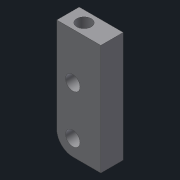
# Autodesk Inventor part: pci_slot_adapter_04
Saved by Autodesk Inventor 2022 (Build 260153000, 153)
## iProperties
Created: 2025-02-02
Part Number: pci_slot_adapter_04
Material: 一般
Document SubType Name: Modeling
Designer: nyxeon
Density: 1 g/cm^3
Appearance: 既定
Author: nyxeon
Autodesk Inventor part; units mm, degrees
ref_plane "YZ Plane" through (0, 0, 0) normal (1, 0, 0) x (0, 1, 0)
ref_plane "XZ Plane" through (0, 0, 0) normal (0, 1, 0) x (-1, 0, 0)
ref_plane "XY Plane" through (0, 0, 0) normal (0, 0, 1) x (1, 0, 0)
sketch "スケッチ1" plane through (0, 0, 0) normal (0, 0, 1) x (1, 0, 0)
  circle A0 centre (250, 70) radius 2.1 construction
  circle A1 centre (250, 85) radius 2.1 construction
  line L0 (258.724, 99.45) -> (245, 99.45) projected
  arc A2 (245, 70) -> (250, 65) centre (250, 70) ccw
  line L1 (245, 70) -> (245, 99.45)
  line L2 (258.724, 99.45) -> (258.724, 65)
  line L3 (258.724, 65) -> (250, 65)
  circle A3 centre (250, 70) radius 2.25
  circle A4 centre (250, 85) radius 2.25
  point P0 (0, 0)
  dimension "d0" = 4.5
  constraints: 6 end point, 3 centre point, 3 coincident, 2 point on circle, 2 tangent, 2 vertical, 1 equal radius, 1 perpendicular
  measures "d0" diameter of A3
extrude "押し出し1" add sketch "スケッチ1" along normal blind 7
sketch "スケッチ2" plane through (245, 99.45, 0) normal (0, 1, 0) x (1, 0, 0)
  circle A0 centre (5, -3.5) radius 1.65 construction
  circle A1 centre (5, -3.5) radius 2.25
  point P0 (-245, 0)
  dimension "d3" = 4.5
  constraints: 1 centre point, 1 coincident
  measures "d3" diameter of A1
extrude "押し出し2" cut sketch "スケッチ2" against normal blind 6
